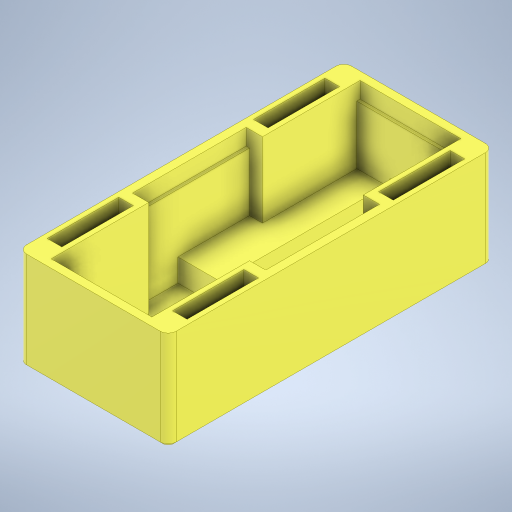
# Autodesk Inventor part: hodinky1
Saved by Autodesk Inventor 2023.2 (Build 272271000, 271)
## iProperties
Created: 2024-01-21
Part Number: hodinky1
Material: Generic
Document SubType Name: Modeling
Designer: marek
Density: 1 g/cm^3
Appearance: Smooth - Yellow
Author: marek
Autodesk Inventor part; units mm, degrees
ref_plane "YZ Plane" through (0, 0, 0) normal (1, 0, 0) x (0, 1, 0)
ref_plane "XZ Plane" through (0, 0, 0) normal (0, 1, 0) x (-1, 0, 0)
ref_plane "XY Plane" through (0, 0, 0) normal (0, 0, 1) x (1, 0, 0)
sketch "Sketch1" plane through (0, 0, 0) normal (0, 1, 0) x (-1, 0, 0)
  line L0 (23, 50) -> (-23, 50)
  line L1 (-23, 50) -> (-23, -50)
  line L2 (-23, -50) -> (23, -50)
  line L3 (23, -50) -> (23, 50)
  line L4 (0, -70) -> (0, 70) projected
  line L5 (-32.2, 0) -> (32.2, 0) projected
  point P0 (0, 0)
  dimension "d0" = 46
  dimension "d1" = 100
  constraints: 8 end point, 2 parallel, 1 horizontal, 1 perpendicular, 2 other
  measures "d0" distance of L2.end L1.end
  measures "d1" distance of L1.end L0.end
extrude "Extrusion1" add sketch "Sketch1" along normal blind 0.5
sketch "Sketch2" plane through (0, 0.5, 0) normal (0, 1, 0) x (1, 0, 0)
  line L0 (-23, 50) -> (-23, -50) projected
  line L1 (23, -50) -> (23, 50) projected
  line L2 (-23, -50) -> (23, -50)
  line L3 (23, -50) -> (23, 50)
  line L4 (23, 50) -> (-23, 50)
  line L5 (-23, 50) -> (-23, -50)
  line L6 (-20.5, -47.5) -> (20.5, -47.5)
  line L7 (20.5, -47.5) -> (20.5, 47.5)
  line L8 (20.5, 47.5) -> (-20.5, 47.5)
  line L9 (-20.5, 47.5) -> (-20.5, -47.5)
  point P0 (0, 0)
  point P1 (23, -50)
  dimension "d4" = 2.5
  dimension "d5" = 2.5
  dimension "d6" = 2.5
  dimension "d7" = 2.5
  constraints: 16 end point, 4 parallel, 2 horizontal, 2 perpendicular
  measures "d4" distance between parallel lines of L0 L9
  measures "d5" distance between parallel lines of L1 L7
  measures "d6" distance between parallel lines of L2 L6
  measures "d7" distance between parallel lines of L4 L8
extrude "Extrusion2" add sketch "Sketch2" along normal blind 30
fillet "Fillet3" radius 2.5 4 edges at (23, 15.25, 50) (-23, 15.25, 50) (23, 15.25, -50) (-23, 15.25, -50)
chamfer "Chamfer8" distance 1 angle 45 8 edges at (0, 0, 50) (22.2678, 0, 49.2678) (23, 0, 0) (22.2678, 0, -49.2678) (0, 0, -50) (-22.2678, 0, -49.2678) (-23, 0, 0) (-22.2678, 0, 49.2678)
sketch "Sketch6" plane through (0, 0.5, 0) normal (0, 1, 0) x (1, 0, 0)
  line L0 (20.5, 47.5) -> (-20.5, 47.5) projected
  line L1 (20.5, -47.5) -> (20.5, 47.5) projected
  line L2 (-20.5, 47.5) -> (20.5, 47.5)
  line L3 (20.5, 47.5) -> (20.5, -47.5)
  line L4 (20.5, -47.5) -> (-20.5, -47.5)
  line L5 (-20.5, -47.5) -> (-20.5, 47.5)
  line L6 (-19.5, -46.5) -> (19.5, -46.5)
  line L7 (19.5, -46.5) -> (19.5, 46.5)
  line L8 (19.5, 46.5) -> (-19.5, 46.5)
  line L9 (-19.5, 46.5) -> (-19.5, -46.5)
  point P0 (0, 0)
  dimension "d39" = 1
  constraints: 16 end point, 4 parallel, 2 perpendicular, 1 horizontal, 3 other
  measures "d39" distance between parallel lines of L4 L6
extrude "Extrusion3" add sketch "Sketch6" along normal blind 25
sketch "Sketch9" plane through (0, 0.5, 0) normal (0, 1, 0) x (1, 0, 0)
  line L0 (0, 70) -> (0, -70) projected
  line L1 (32.2, 0) -> (-32.2, 0) projected
  line L2 (7.5, -39.7) -> (-7.5, -39.7)
  line L3 (-7.5, -39.7) -> (-7.5, -26.7)
  line L4 (-7.5, -26.7) -> (7.5, -26.7)
  line L5 (7.5, -26.7) -> (7.5, -39.7)
  line L6 (19.5, -46.5) -> (-19.5, -46.5) projected
  point P0 (0, 0)
  point P1 (7.5, -33.2)
  dimension "d52" = 13
  dimension "d94" = 6.8
  dimension "d114" = 15
  constraints: 8 end point, 2 parallel, 1 horizontal, 1 midpoint, 1 perpendicular, 1 other
  measures "d52" distance of L2.end L3.end
  measures "d94" distance between parallel lines of L6 L2
  measures "d114" distance from line of point (7.5, -33.2) L3
extrude "MAX30102" cut sketch "Sketch9" against normal up to surface (0.5 mm away)
sketch "Sketch20" plane through (0, 0.5, 0) normal (0, 1, 0) x (1, 0, 0)
  line L0 (19.5, 46.5) -> (19.5, -46.5) projected
  line L1 (19.5, -46.5) -> (-19.5, -46.5) projected
  line L2 (15.5, -17.5) -> (20.5, -17.5)
  line L3 (20.5, -17.5) -> (20.5, -47.5)
  line L4 (20.5, -47.5) -> (15.5, -47.5)
  line L5 (15.5, -47.5) -> (15.5, -17.5)
  line L6 (20.5, -47.5) -> (-20.5, -47.5) projected
  line L7 (20.5, 47.5) -> (20.5, -47.5) projected
  line L8 (20.5, 47.5) -> (20.5, -47.5) projected
  line L9 (20.5, 47.5) -> (15.5, 47.5)
  line L10 (15.5, 47.5) -> (15.5, 17.5)
  line L11 (15.5, 17.5) -> (20.5, 17.5)
  line L12 (20.5, 17.5) -> (20.5, 47.5)
  point P0 (0, 0)
  dimension "d143" = 5
  dimension "d144" = 30
  dimension "d154" = 5
  dimension "d155" = 30
  constraints: 16 end point, 4 parallel, 2 collinear, 2 horizontal, 2 perpendicular
  measures "d143" distance of L3.end L4.end
  measures "d144" distance of L2.end L3.end
  measures "d154" distance of L11.end L10.end
  measures "d155" distance of L9.end L10.end
extrude "Extrusion14" add sketch "Sketch20" along normal up to surface (30 mm away) contours L11 L10 L9 L7 | L2 L3 L4 L5 L1 L0 | L0 L1 L5 L2
sketch "Sketch21" plane through (0, 30.5, 0) normal (0, 1, 0) x (1, 0, 0)
  line L0 (17, -20.7) -> (21.5, -20.7)
  line L1 (21.5, -20.7) -> (21.5, -42.7)
  line L2 (21.5, -42.7) -> (17, -42.7)
  line L3 (17, -42.7) -> (17, -20.7)
  line L4 (15.5, -47.5) -> (15.5, -17.5) projected
  line L5 (-20.5, -50) -> (20.5, -50) projected
  line L6 (17, 42.7) -> (21.5, 42.7)
  line L7 (21.5, 42.7) -> (21.5, 20.7)
  line L8 (21.5, 20.7) -> (17, 20.7)
  line L9 (17, 20.7) -> (17, 42.7)
  line L10 (15.5, 17.5) -> (15.5, 47.5) projected
  line L11 (20.5, 50) -> (-20.5, 50) projected
  point P0 (0, 0)
  dimension "d147" = 4.5
  dimension "d149" = 1.5
  dimension "d152" = 22
  dimension "d153" = 7.3
  dimension "d156" = 4.5
  dimension "d157" = 22
  dimension "d158" = 1.5
  dimension "d159" = 7.3
  constraints: 16 end point, 4 parallel, 2 horizontal, 2 perpendicular
  measures "d147" distance of L1.end L2.end
  measures "d149" distance between parallel lines of L4 L3
  measures "d152" distance of L0.end L1.end
  measures "d153" distance between parallel lines of L5 L2
  measures "d156" distance of L7.end L8.end
  measures "d157" distance of L6.end L7.end
  measures "d158" distance between parallel lines of L10 L9
  measures "d159" distance between parallel lines of L11 L6
extrude "Extrusion15" cut sketch "Sketch21" against normal up to surface (30.5 mm away)
mirror "Mirror2" about plane through (0, 0, 0) normal (1, 0, 0) of "Extrusion15", "Extrusion14"
sketch "Sketch24" plane through (0, 0.5, 0) normal (0, 1, 0) x (1, 0, 0)
  line L0 (15.5, 17.5) -> (15.5, 47.5) projected
  line L1 (15.5, -4.5) -> (6.5, -4.5)
  line L2 (6.5, -4.5) -> (6.5, 46.5)
  line L3 (6.5, 46.5) -> (15.5, 46.5)
  line L4 (15.5, 46.5) -> (15.5, 17.5)
  line L5 (-15.5, 46.5) -> (15.5, 46.5) projected
  line L6 (-15.5, 46.5) -> (-6.5, 46.5)
  line L7 (-6.5, 46.5) -> (-6.5, -4.5)
  line L8 (-6.5, -4.5) -> (-15.5, -4.5)
  line L9 (-15.5, 17.5) -> (-15.5, 46.5)
  line L10 (-19.5, -17.5) -> (-19.5, 17.5) projected
  line L11 (-15.5, -4.5) -> (-19.5, -4.5)
  line L12 (-19.5, -4.5) -> (-19.5, 17.5)
  line L13 (-19.5, 17.5) -> (-15.5, 17.5)
  line L14 (20.5, 17.5) -> (15.5, 17.5) projected
  line L15 (19.5, 17.5) -> (19.5, -17.5) projected
  line L16 (15.5, 17.5) -> (19.5, 17.5)
  line L17 (19.5, 17.5) -> (19.5, -4.5)
  line L18 (19.5, -4.5) -> (15.5, -4.5)
  point P0 (0, 0)
  dimension "d164" = 51
  dimension "d166" = 51
  dimension "d173" = 9
  dimension "d174" = 9
  constraints: 28 end point, 6 parallel, 4 horizontal, 4 perpendicular, 3 point on line, 1 collinear
  measures "d164" distance of L1.end L2.end
  measures "d166" distance of L6.end L7.end
  measures "d173" distance between parallel lines of L9 L7
  measures "d174" distance between parallel lines of L0 L2
extrude "Extrusion16" add sketch "Sketch24" along normal blind 7
sketch "Sketch23" plane through (20.5, 30.5, -50) normal (0, 0, -1) x (-1, 0, 0)
  line L0 (15, -20.5) -> (26, -20.5)
  line L1 (26, -20.5) -> (26, -27.5)
  line L2 (26, -27.5) -> (15, -27.5)
  line L3 (15, -27.5) -> (15, -20.5)
  line L4 (20.5, -36.6) -> (20.5, 6.1) projected
  line L5 (-11.7, -30.5) -> (52.7, -30.5) projected
  line L6 (5, -30) -> (36, -30) projected
  point P0 (20.5, -30.5)
  point P1 (27, -23)
  dimension "d160" = 11
  dimension "d161" = 7
  dimension "d172" = 4.5
  constraints: 6 end point, 2 horizontal, 2 parallel, 1 vertical, 3 other
  measures "d160" distance of L2.start L2.end
  measures "d161" distance of L0.end L2.start
  measures "d172" distance from line of L2 point (27, -23)
extrude "Extrusion17" cut sketch "Sketch23" against normal blind 5
fillet "Face Fillet1" radius 0.5 1 edges at (5.5, 10, -48.25)
fillet "Face Fillet2" radius 0.5 1 edges at (5.5, 3, -48.25)
fillet "Face Fillet3" radius 0.5 1 edges at (-5.5, 3, -48.25)
fillet "Face Fillet4" radius 0.5 1 edges at (-5.5, 10, -48.25)
fillet "Face Fillet5" radius 0.5 1 edges at (-7.5, 0.25, 39.7)
fillet "Face Fillet6" radius 0.5 1 edges at (7.5, 0.25, 39.7)
fillet "Face Fillet7" radius 0.5 1 edges at (-7.5, 0.25, 26.7)
fillet "Face Fillet8" radius 0.5 1 edges at (7.5, 0.25, 26.7)
body "Solid1"
